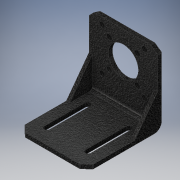
# Autodesk Inventor part: Stepper Bracket
Saved by Autodesk Inventor 2018 (Build 220112000, 112)
## iProperties
Created: 2018-03-28
Part Number: Stepper Bracket
Material: Generic
Document SubType Name: Modeling
Designer: Ajith Thomas
Density: 1 g/cm^3
Appearance: Default
Author: Ajith Thomas
Autodesk Inventor part; units mm, degrees
ref_plane "YZ Plane" through (0, 0, 0) normal (1, 0, 0) x (0, 1, 0)
ref_plane "XZ Plane" through (0, 0, 0) normal (0, 1, 0) x (-1, 0, 0)
sketch "Sketch1" plane through (0, 0, 0) normal (1, 0, 0) x (0, 1, 0)
  line L0 (0, 0) -> (0, -22.65)
  line L1 (0, 0) -> (0, 26.65)
  line L2 (4, -26.65) -> (51, -26.65)
  arc A0 (0, -22.65) -> (4, -26.65) centre (4, -22.65) ccw
  point P0 (0, -26.65)
  dimension "d0" = 26.65
  dimension "d1" = 26.65
  dimension "d2" = 51
  dimension "d3" = 4
  constraints: 6 end point, 2 point on circle, 2 point on line, 2 tangent, 2 vertical, 1 centre point, 1 horizontal
  measures "d0" distance of L0.start point (0, -26.65)
  measures "d1" distance of L0.start L1.end
  measures "d2" distance of point (0, -26.65) L2.end
  measures "d3" radius of A0
ref_plane "Work Plane1" through (0, 0, 26.65) normal (0, 0, 1) x (1, 0, 0)
sketch "Sketch2" plane through (0, 0, 26.65) normal (0, 0, 1) x (1, 0, 0)
  line L0 (-25, 1.5) -> (25, 1.5)
  line L1 (25, 1.5) -> (25, -1.5)
  line L2 (25, -1.5) -> (-25, -1.5)
  line L3 (-25, -1.5) -> (-25, 1.5)
  line L4 (-25, 1.5) -> (25, -1.5) construction
  line L5 (25, 1.5) -> (-25, -1.5) construction
  point P0 (0, 0)
  dimension "d4" = 50
  dimension "d5" = 3
  constraints: 12 end point, 2 midpoint, 2 parallel, 1 horizontal, 1 perpendicular
  measures "d4" distance of L1.end L2.end
  measures "d5" distance of L0.end L1.end
sweep "Sweep1" add profiles "Sketch2" path "Sketch1"
sketch "Sketch3" plane through (25, 4, -28.15) normal (0, 0, -1) x (-1, 0, 0)
  line L0 (0, 47) -> (50, 47) construction
  line L1 (50, 0) -> (50, 47) construction
  circle A0 centre (25, 26.5) radius 11
  point P0 (25, -4)
  dimension "d8" = 22
  dimension "d9" = 20.5
  dimension "d10" = 25
  constraints: 1 centre point
  measures "d8" diameter of A0
  measures "d9" distance from line of L0 A0.centre
  measures "d10" distance from line of L1 A0.centre
extrude "Extrusion1" cut sketch "Sketch3" against normal blind 10
sketch "Sketch4" plane through (25, 4, -28.15) normal (0, 0, -1) x (-1, 0, 0)
  circle A0 centre (25, 26.5) radius 11 construction
  line L0 (50, 0) -> (50, 47) construction
  line L1 (0, 0) -> (0, 47) construction
  line L2 (0, 47) -> (50, 47) construction
  line L3 (0, 0) -> (50, 0) construction
  circle A1 centre (40.5, 42) radius 2
  line L4 (25, 26.5) -> (14, 26.5) construction
  circle A2 centre (25, 26.5) radius 11 construction
  line L5 (25, 26.5) -> (25, 15.5) construction
  circle A3 centre (9.5, 42) radius 2
  circle A4 centre (40.5, 11) radius 2
  circle A5 centre (9.5, 11) radius 2
  line L6 (25, 26.5) -> (40.5, 42) construction
  circle A6 centre (35.253, 36.753) radius 2
  circle A7 centre (14.747, 36.753) radius 2
  circle A8 centre (35.253, 16.247) radius 2
  circle A9 centre (14.747, 16.247) radius 2
  point P0 (25, -4)
  point P1 (33.8388, 35.3388)
  point P2 (32.7782, 34.2782)
  dimension "d17" = 4
  dimension "d13" = 4
  dimension "d14" = 15.5
  dimension "d15" = 15.5
  dimension "d18" = 1.5
  constraints: 7 centre point, 6 end point, 6 symmetric about line, 3 point on circle, 3 point on line, 1 horizontal, 1 perpendicular, 9 other
  measures "d13" diameter of A1
  measures "d14" horizontal distance of L6.end L4.start
  measures "d15" horizontal distance of L4.start L6.end
  measures "d18" distance of point (33.839, 35.339) point (32.778, 34.278)
extrude "Extrusion2" cut sketch "Sketch4" against normal blind 10
sketch "Sketch5" plane through (25, 4, -28.15) normal (0, 0, -1) x (-1, 0, 0)
  line L0 (0, 47) -> (50, 47) construction
  line L1 (50, 0) -> (50, 47) construction
  line L2 (0, 0) -> (0, 47) construction
  line L3 (0, 43.5) -> (5, 47)
  line L4 (25, 47) -> (25, 37.5) construction
  circle A0 centre (25, 26.5) radius 11 construction
  line L5 (50, 43.5) -> (45, 47)
  line L6 (0, 43.5) -> (0, 47)
  line L7 (0, 47) -> (5, 47)
  line L8 (45, 47) -> (50, 47)
  line L9 (50, 47) -> (50, 43.5)
  line L10 (50, 0) -> (50, 47) projected
  point P0 (25, -4)
  point P1 (0, 23.5)
  dimension "d21" = 20
  dimension "d22" = 20
  constraints: 14 end point, 4 collinear, 2 midpoint, 2 point on line, 2 symmetric about line, 1 vertical, 1 vertical alignment, 1 other
  measures "d21" distance of L3.end L4.start
  measures "d22" distance of L3.start point (0, 23.5)
extrude "Extrusion3" cut sketch "Sketch5" against normal blind 10
sketch "Sketch6" plane through (-25, 1.5, 26.65) normal (0, 1, 0) x (1, 0, 0)
  line L0 (0, 0) -> (0, 49.3) construction
  line L1 (0, 0) -> (50, 0) construction
  line L2 (50, 0) -> (50, 49.3) construction
  line L3 (45, 0) -> (50, 4.65)
  line L4 (25, 0) -> (25, 26.65) construction
  line L5 (5, 0) -> (0, 4.65)
  line L6 (5, 0) -> (0, 0)
  line L7 (0, 4.65) -> (0, 0)
  line L8 (45, 0) -> (50, 0)
  line L9 (50, 4.65) -> (50, 0)
  point P0 (50, 24.65)
  dimension "d25" = 20
  dimension "d26" = 20
  constraints: 14 end point, 2 collinear, 2 midpoint, 2 point on line, 2 symmetric about line, 2 vertical, 1 perpendicular
  measures "d25" distance of L4.start L3.start
  measures "d26" distance of point (50, 24.65) L3.end
extrude "Extrusion4" cut sketch "Sketch6" against normal blind 10
sketch "Sketch7" plane through (-25, 1.5, -22.65) normal (0, 1, 0) x (1, 0, 0)
  line L0 (10, -40.3) -> (10, -6.3) construction
  line L1 (12, -38.3) -> (12, -8.3)
  line L2 (8, -8.3) -> (8, -38.3)
  arc A0 (8, -38.3) -> (12, -38.3) centre (10, -38.3) ccw
  arc A1 (12, -8.3) -> (8, -8.3) centre (10, -8.3) ccw
  line L3 (11.5, 2.5) -> (7.5, 2.5) construction
  line L4 (0, -44.65) -> (0, 0) construction
  line L5 (45, -49.3) -> (5, -49.3) construction
  line L6 (25, -49.3) -> (25, -22.65) construction
  line L7 (38, -38.3) -> (38, -8.3)
  line L8 (42, -8.3) -> (42, -38.3)
  arc A2 (38, -38.3) -> (42, -38.3) centre (40, -38.3) ccw
  arc A3 (42, -8.3) -> (38, -8.3) centre (40, -8.3) ccw
  point P0 (10, -23.3)
  dimension "d29" = 34
  dimension "d30" = 4
  dimension "d31" = 8
  dimension "d32" = 9
  constraints: 14 end point, 10 point on circle, 6 symmetric about line, 4 centre point, 4 tangent, 2 midpoint, 2 point on line, 2 vertical, 1 parallel, 2 other
  measures "d29" distance of L0.start L0.end
  measures "d30" diameter of A1
  measures "d31" distance between parallel lines of L4 L2
  measures "d32" distance from line of L5 L0.start
extrude "Extrusion5" cut sketch "Sketch7" against normal blind 10
fillet "Fillet1" radius 1 8 edges at (20, 51, -26.65) (-20, 51, -26.65) (-25, 47.5, -26.65) (25, 47.5, -26.65) (25, 0, 22) (20, 0, 26.65) (-20, 0, 26.65) (-25, 0, 22)
sketch "Sketch8" plane through (-25, 4, -25.15) normal (-1, 0, 0) x (0, 0, 1)
  line L0 (0, 0) -> (0, 42.9793) projected
  arc A0 (0, 0) -> (2.5, -2.5) centre (2.5, 0) ccw projected
  line L1 (46.7144, -2.5) -> (2.5, -2.5) projected
  line L2 (10.8, -2.5) -> (40.8, -2.5) projected
  line L3 (0, 19.9793) -> (16.7144, -2.5)
  point P0 (25.15, -4)
  dimension "d36" = 30
  dimension "d37" = 23
  constraints: 2 end point, 2 point on line
  measures "d36" distance of L1.start L3.end
  measures "d37" distance of L0.end L3.start
extrude "Extrusion6" add sketch "Sketch8" against normal blind 2.5
mirror "Mirror1" about plane through (0, 0, 0) normal (1, 0, 0) of "Extrusion6"
body "Solid1"
